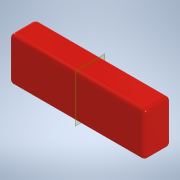
# Autodesk Inventor part: аккум
Saved by Autodesk Inventor 2021.1 (Build 251245010, 245A)
## iProperties
Created: 2023-02-11
Part Number: аккум
Material: Типовые
Document SubType Name: Modeling
Designer: zmoze
Density: 1 g/cm^3
Appearance: Оранжево-красный
Author: zmoze
Autodesk Inventor part; units mm, degrees
ref_plane "YZ Plane" through (0, 0, 0) normal (1, 0, 0) x (0, 1, 0)
ref_plane "XZ Plane" through (0, 0, 0) normal (0, 1, 0) x (-1, 0, 0)
ref_plane "XY Plane" through (0, 0, 0) normal (0, 0, 1) x (1, 0, 0)
sketch "Эскиз1" plane through (0, 0, 0) normal (0, 0, 1) x (1, 0, 0)
  line L0 (0, 0) -> (106, 0)
  line L1 (106, 0) -> (106, 34)
  line L2 (106, 34) -> (0, 34)
  line L3 (0, 34) -> (0, 0)
  dimension "d0" = 106
  dimension "d1" = 34
  constraints: 8 end point, 2 parallel, 1 horizontal, 1 perpendicular
  measures "d0" distance of L1.end L2.end
  measures "d1" distance of L0.end L1.end
extrude "Выдавливание1" add sketch "Эскиз1" along normal blind 21
fillet "Сопряжение1" radius 3 12 edges at (106, 34, 10.5) (106, 17, 21) (53, 34, 21) (53, 34, 0) (0, 34, 10.5) (106, 17, 0) (106, 0, 10.5) (0, 17, 21) (0, 0, 10.5) (0, 17, 0) (53, 0, 0) (53, 0, 21)
ref_plane "РабПлоскость1" through (53, 3, 3) normal (-1, 0, 0) x (0, 0, 1)
